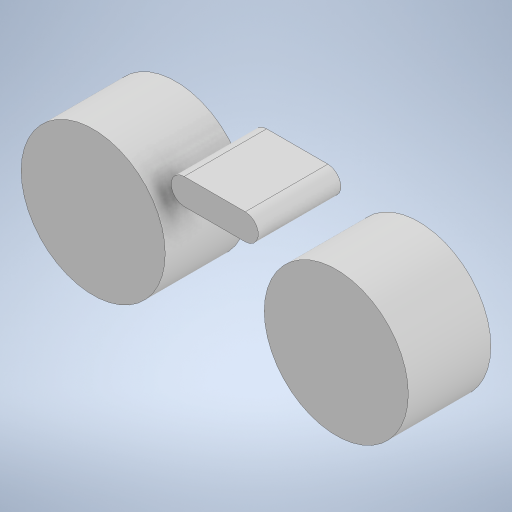
# Autodesk Inventor part: Sonar
Saved by Autodesk Inventor 2024.1 (Build 281209000, 209)
## iProperties
Created: 2024-05-13
Part Number: Sonar
Material: Generic
Document SubType Name: Modeling
Designer: cyan924
Density: 1 g/cm^3
Appearance: Default
Author: cyan924
Autodesk Inventor part; units mm, degrees
(part 1 of 2)
ref_plane "YZ Plane" through (0, 0, 0) normal (1, 0, 0) x (0, 1, 0)
ref_plane "XZ Plane" through (0, 0, 0) normal (0, 1, 0) x (-1, 0, 0)
ref_plane "XY Plane" through (0, 0, 0) normal (0, 0, 1) x (1, 0, 0)
sketch "Sketch1" plane through (0, 0, 0) normal (0, 0, 1) x (1, 0, 0)
  line L0 (-74.4703, -18.8519) -> (-29.4703, -18.8519)
  line L1 (-29.4703, -18.8519) -> (-29.4703, -38.8519)
  line L2 (-29.4703, -38.8519) -> (-74.4703, -38.8519)
  line L3 (-74.4703, -38.8519) -> (-74.4703, -18.8519)
  circle A0 centre (-65.4703, -28.8519) radius 8
  circle A1 centre (-38.4703, -28.8519) radius 8
  arc A2 (-48.5719, -23.254) -> (-48.5719, -20.3658) centre (-48.5719, -21.8099) ccw
  line L4 (-55.3687, -20.3658) -> (-48.5719, -20.3658)
  arc A3 (-55.3687, -20.3658) -> (-55.3687, -23.254) centre (-55.3687, -21.8099) ccw
  line L5 (-48.5719, -23.254) -> (-55.3687, -23.254)
  circle A4 centre (-38.4703, -28.8519) radius 7 construction
  line L6 (-53.2518, -34.5647) -> (-53.3871, -34.5647) construction
  line L7 (-53.3871, -34.5647) -> (-53.3871, -34.4697) construction
  line L8 (-53.3871, -34.4697) -> (-52.7733, -34.4697) construction
  spline S0 degree 3 poles (-52.7733, -34.4697) (-52.7602, -34.4698) (-52.735, -34.47) (-52.6985, -34.4711) (-52.6648, -34.4736) (-52.6337, -34.4764) (-52.6054, -34.4804) (-52.5798, -34.4853) (-52.5569, -34.4908) (-52.5428, -34.4956) (-52.5361, -34.4979) knots 0 0 0 0 0.163445 0.315489 0.456291 0.585864 0.705429 0.813371 0.911718 1 1 1 1 construction
  spline S1 degree 3 poles (-52.5361, -34.4979) (-52.5274, -34.5013) (-52.5103, -34.508) (-52.486, -34.5204) (-52.4632, -34.5344) (-52.4419, -34.5504) (-52.4222, -34.5683) (-52.4038, -34.5876) (-52.3872, -34.609) (-52.3723, -34.6321) (-52.3587, -34.6564) (-52.347, -34.6821) (-52.3373, -34.7092) (-52.3292, -34.7374) (-52.3228, -34.7668) (-52.3185, -34.7974) (-52.3156, -34.8291) (-52.3153, -34.8508) (-52.3152, -34.8617) knots 0 0 0 0 0.061377 0.120918 0.179441 0.23763 0.295967 0.354252 0.413289 0.473845 0.53511 0.596983 0.659861 0.724251 0.789992 0.857734 0.927822 1 1 1 1 construction
  spline S2 degree 3 poles (-52.3152, -34.8617) (-52.3155, -34.8777) (-52.316, -34.9089) (-52.3215, -34.9545) (-52.3302, -34.9977) (-52.3427, -35.0381) (-52.3582, -35.0754) (-52.3759, -35.1093) (-52.3962, -35.1395) (-52.4194, -35.1668) (-52.4469, -35.1914) (-52.4793, -35.2145) (-52.5171, -35.2368) (-52.5449, -35.2498) (-52.5594, -35.2567) knots 0 0 0 0 0.096488 0.188417 0.276865 0.362159 0.443456 0.520182 0.592724 0.662929 0.735428 0.814887 0.903064 1 1 1 1 construction
  line L9 (-52.5594, -35.2567) -> (-52.5594, -35.1617) construction
  spline S3 degree 3 poles (-52.5594, -35.1617) (-52.5473, -35.1541) (-52.5236, -35.1391) (-52.4929, -35.1113) (-52.4668, -35.0805) (-52.4457, -35.0462) (-52.4295, -35.0082) (-52.4182, -34.9661) (-52.4114, -34.9198) (-52.4106, -34.8876) (-52.4101, -34.8708) knots 0 0 0 0 0.124736 0.243843 0.35972 0.474789 0.593462 0.719307 0.853832 1 1 1 1 construction
  spline S4 degree 3 poles (-52.4101, -34.8708) (-52.4106, -34.8543) (-52.4114, -34.8223) (-52.4182, -34.7764) (-52.4295, -34.7345) (-52.4457, -34.6969) (-52.4652, -34.664) (-52.4867, -34.6354) (-52.5113, -34.6124) (-52.5339, -34.5969) (-52.554, -34.5873) (-52.5714, -34.5812) (-52.5909, -34.5762) (-52.6127, -34.572) (-52.6368, -34.5686) (-52.6632, -34.5664) (-52.6917, -34.5648) (-52.7115, -34.5647) (-52.7218, -34.5647) knots 0 0 0 0 0.09818 0.189281 0.274487 0.355219 0.431123 0.501038 0.566565 0.629684 0.662677 0.698735 0.738584 0.782147 0.830394 0.882567 0.939223 1 1 1 1 construction
  line L10 (-52.7218, -34.5647) -> (-52.7619, -34.5647) construction
  spline S5 degree 3 poles (-52.7619, -34.5647) (-52.7504, -34.5743) (-52.7277, -34.5935) (-52.6978, -34.6264) (-52.6724, -34.6626) (-52.6513, -34.7015) (-52.6346, -34.7426) (-52.6224, -34.7852) (-52.6149, -34.8291) (-52.6141, -34.8588) (-52.6137, -34.8738) knots 0 0 0 0 0.126584 0.250941 0.374443 0.499573 0.624733 0.748994 0.873157 1 1 1 1 construction
  spline S6 degree 3 poles (-52.6137, -34.8738) (-52.6139, -34.8826) (-52.6142, -34.9002) (-52.6165, -34.9264) (-52.6209, -34.952) (-52.6265, -34.9773) (-52.634, -35.0021) (-52.6429, -35.0267) (-52.6537, -35.0507) (-52.666, -35.0743) (-52.6797, -35.0968) (-52.6946, -35.1183) (-52.7105, -35.1385) (-52.7276, -35.1574) (-52.746, -35.1748) (-52.7653, -35.191) (-52.7859, -35.2058) (-52.8075, -35.2194) (-52.83, -35.2312) (-52.8531, -35.2416) (-52.8767, -35.2506) (-52.9009, -35.2578) (-52.9256, -35.2633) (-52.9509, -35.2674) (-52.9767, -35.2697) (-52.9941, -35.2701) (-53.0029, -35.2702) knots 0 0 0 0 0.042863 0.085187 0.127219 0.169041 0.210896 0.252856 0.295658 0.338581 0.38149 0.423606 0.465089 0.506333 0.547059 0.587693 0.628691 0.669961 0.711048 0.752006 0.792681 0.833453 0.874196 0.915497 0.95748 1 1 1 1 construction
  spline S7 degree 3 poles (-53.0029, -35.2702) (-53.0117, -35.2701) (-53.0292, -35.2698) (-53.0552, -35.2671) (-53.0808, -35.2632) (-53.1058, -35.2571) (-53.1305, -35.2497) (-53.1546, -35.2406) (-53.1783, -35.2297) (-53.2015, -35.2173) (-53.2239, -35.2033) (-53.2452, -35.1881) (-53.2651, -35.1714) (-53.284, -35.1536) (-53.3017, -35.1345) (-53.318, -35.114) (-53.3333, -35.0924) (-53.3473, -35.0696) (-53.3596, -35.046) (-53.3709, -35.022) (-53.3798, -34.9975) (-53.3877, -34.9729) (-53.3932, -34.9478) (-53.3975, -34.9224) (-53.4001, -34.8967) (-53.4005, -34.8795) (-53.4006, -34.8708) knots 0 0 0 0 0.042034 0.083905 0.125069 0.166158 0.20721 0.248491 0.289878 0.33217 0.374476 0.416225 0.45761 0.499073 0.540553 0.582249 0.62455 0.667433 0.710323 0.752467 0.794065 0.835216 0.876228 0.917446 0.958643 1 1 1 1 construction
  spline S8 degree 3 poles (-53.4006, -34.8708) (-53.4002, -34.8566) (-53.3994, -34.8285) (-53.3931, -34.7872) (-53.3829, -34.7473) (-53.3684, -34.7086) (-53.3486, -34.6708) (-53.3225, -34.6341) (-53.2898, -34.5983) (-53.2648, -34.5762) (-53.2518, -34.5647) knots 0 0 0 0 0.120911 0.238762 0.354755 0.470359 0.589144 0.716329 0.852445 1 1 1 1 construction
  line L11 (-50.2203, -36.6833) -> (-51.2787, -36.6833) construction
  line L12 (-51.2787, -36.6833) -> (-51.2787, -36.0862) construction
  line L13 (-51.2787, -36.0862) -> (-51.1701, -36.0862) construction
  line L14 (-51.1701, -36.0862) -> (-51.1701, -36.5883) construction
  line L15 (-51.1701, -36.5883) -> (-50.8445, -36.5883) construction
  line L16 (-50.8445, -36.5883) -> (-50.8445, -36.0862) construction
  line L17 (-50.8445, -36.0862) -> (-50.7359, -36.0862) construction
  line L18 (-50.7359, -36.0862) -> (-50.7359, -36.5883) construction
  line L19 (-50.7359, -36.5883) -> (-50.3289, -36.5883) construction
  line L20 (-50.3289, -36.5883) -> (-50.3289, -36.0862) construction
  line L21 (-50.3289, -36.0862) -> (-50.2203, -36.0862) construction
  line L22 (-50.2203, -36.0862) -> (-50.2203, -36.6833) construction
  spline S9 degree 3 poles (-51.0073, -35.5176) (-51.007, -35.505) (-51.0065, -35.4797) (-51.0018, -35.4422) (-50.9947, -35.4053) (-50.9843, -35.3696) (-50.9716, -35.3355) (-50.9573, -35.3037) (-50.9411, -35.2746) (-50.923, -35.248) (-50.9024, -35.2238) (-50.8795, -35.2016) (-50.8542, -35.1811) (-50.8355, -35.1695) (-50.826, -35.1636) knots 0 0 0 0 0.091262 0.182067 0.271888 0.362021 0.450031 0.533934 0.613304 0.689893 0.765431 0.841449 0.919739 1 1 1 1 construction
  line L23 (-50.826, -35.1636) -> (-50.7766, -35.2431) construction
  spline S10 degree 3 poles (-50.7766, -35.2431) (-50.7875, -35.2518) (-50.8088, -35.269) (-50.8363, -35.2988) (-50.8599, -35.3305) (-50.8792, -35.3648) (-50.8941, -35.4015) (-50.9046, -35.4405) (-50.9112, -35.4818) (-50.9119, -35.5101) (-50.9123, -35.5246) knots 0 0 0 0 0.128324 0.252584 0.373506 0.493364 0.614609 0.73847 0.865995 1 1 1 1 construction
  spline S11 degree 3 poles (-50.9123, -35.5246) (-50.912, -35.5362) (-50.9114, -35.5591) (-50.9074, -35.5926) (-50.9003, -35.6246) (-50.8909, -35.6551) (-50.8782, -35.6841) (-50.8629, -35.7115) (-50.845, -35.7376) (-50.8243, -35.7617) (-50.8018, -35.7837) (-50.7777, -35.8028) (-50.7527, -35.8194) (-50.7262, -35.8324) (-50.6987, -35.8431) (-50.6698, -35.8501) (-50.6399, -35.8548) (-50.6195, -35.8553) (-50.6091, -35.8556) knots 0 0 0 0 0.069522 0.136921 0.201969 0.265462 0.328248 0.390817 0.45355 0.517542 0.580738 0.641922 0.701597 0.760313 0.818757 0.877718 0.938094 1 1 1 1 construction
  spline S12 degree 3 poles (-50.6091, -35.8556) (-50.5956, -35.855) (-50.5687, -35.854) (-50.5289, -35.8457) (-50.4906, -35.8318) (-50.4538, -35.8131) (-50.4198, -35.7894) (-50.3893, -35.7615) (-50.3628, -35.7295) (-50.3409, -35.6936) (-50.3233, -35.6547) (-50.3108, -35.6131) (-50.3032, -35.5693) (-50.3022, -35.5393) (-50.3017, -35.524) knots 0 0 0 0 0.080524 0.160375 0.240333 0.322539 0.405033 0.486605 0.567872 0.651338 0.736242 0.821532 0.909006 1 1 1 1 construction
  spline S13 degree 3 poles (-50.3017, -35.524) (-50.3021, -35.51) (-50.3029, -35.4824) (-50.3094, -35.4422) (-50.3201, -35.4038) (-50.3349, -35.3674) (-50.3541, -35.333) (-50.3778, -35.3009) (-50.4053, -35.2703) (-50.4266, -35.2523) (-50.4374, -35.2431) knots 0 0 0 0 0.129981 0.255447 0.377298 0.498442 0.619372 0.741857 0.868564 1 1 1 1 construction
  line L24 (-50.4374, -35.2431) -> (-50.3853, -35.1636) construction
  spline S14 degree 3 poles (-50.3853, -35.1636) (-50.3783, -35.1683) (-50.3645, -35.1777) (-50.345, -35.1935) (-50.3268, -35.2104) (-50.3098, -35.2286) (-50.2937, -35.2476) (-50.2793, -35.2683) (-50.2656, -35.2899) (-50.2533, -35.3126) (-50.2423, -35.3363) (-50.2328, -35.3609) (-50.2246, -35.3863) (-50.2182, -35.4125) (-50.213, -35.4396) (-50.2096, -35.4675) (-50.207, -35.4963) (-50.2068, -35.5157) (-50.2068, -35.5255) knots 0 0 0 0 0.059633 0.119069 0.178197 0.236957 0.295932 0.355856 0.416473 0.477742 0.539903 0.602538 0.665422 0.729765 0.794829 0.861827 0.930011 1 1 1 1 construction
  spline S15 degree 3 poles (-50.2068, -35.5255) (-50.207, -35.5405) (-50.2076, -35.5699) (-50.2134, -35.6129) (-50.2221, -35.6541) (-50.2346, -35.6933) (-50.2511, -35.7305) (-50.2708, -35.7659) (-50.2944, -35.7992) (-50.3212, -35.8301) (-50.3503, -35.8583) (-50.3815, -35.8829) (-50.4142, -35.9037) (-50.4485, -35.9209) (-50.4843, -35.9343) (-50.5218, -35.9436) (-50.5607, -35.9495) (-50.5872, -35.9502) (-50.6007, -35.9506) knots 0 0 0 0 0.069569 0.136355 0.201125 0.264488 0.327183 0.389579 0.452173 0.515875 0.579188 0.640132 0.69999 0.75865 0.817794 0.876966 0.937625 1 1 1 1 construction
  spline S16 degree 3 poles (-50.6007, -35.9506) (-50.6098, -35.9504) (-50.6279, -35.9502) (-50.6549, -35.9471) (-50.6815, -35.9432) (-50.7074, -35.9365) (-50.7329, -35.9288) (-50.7579, -35.919) (-50.7824, -35.9075) (-50.8063, -35.8944) (-50.8293, -35.8797) (-50.851, -35.8634) (-50.8717, -35.8462) (-50.8906, -35.8271) (-50.9086, -35.8072) (-50.9252, -35.7857) (-50.9403, -35.7628) (-50.9544, -35.7389) (-50.9669, -35.7139) (-50.9777, -35.688) (-50.9869, -35.6614) (-50.9942, -35.634) (-51.0003, -35.606) (-51.0041, -35.5772) (-51.0068, -35.5477) (-51.0071, -35.5278) (-51.0073, -35.5176) knots 0 0 0 0 0.041291 0.082136 0.122636 0.162831 0.203007 0.243526 0.284173 0.32541 0.366855 0.407551 0.448187 0.488683 0.529015 0.569843 0.61137 0.653238 0.695446 0.737751 0.780043 0.822807 0.865978 0.909595 0.954231 1 1 1 1 construction
  line L25 (-50.2203, -34.9736) -> (-51.3058, -34.9736) construction
  line L26 (-51.3058, -34.9736) -> (-51.3058, -34.8787) construction
  line L27 (-51.3058, -34.8787) -> (-50.8477, -34.8787) construction
  spline S17 degree 3 poles (-50.8477, -34.8787) (-50.8604, -34.8685) (-50.8852, -34.8486) (-50.9176, -34.8152) (-50.9456, -34.7808) (-50.9682, -34.7446) (-50.9859, -34.7067) (-50.9981, -34.6673) (-51.0059, -34.6263) (-51.0068, -34.5985) (-51.0073, -34.5844) knots 0 0 0 0 0.140704 0.273958 0.400629 0.522804 0.641767 0.760002 0.878421 1 1 1 1 construction
  spline S18 degree 3 poles (-51.0073, -34.5844) (-51.0068, -34.5701) (-51.0058, -34.542) (-50.9972, -34.5014) (-50.9837, -34.4631) (-50.9645, -34.4279) (-50.9407, -34.3961) (-50.9131, -34.3683) (-50.8814, -34.3451) (-50.852, -34.3296) (-50.8258, -34.3195) (-50.8034, -34.313) (-50.7784, -34.3076) (-50.7508, -34.3028) (-50.7206, -34.2997) (-50.6878, -34.2971) (-50.6524, -34.2953) (-50.6279, -34.2953) (-50.6153, -34.2952) knots 0 0 0 0 0.077236 0.151245 0.22342 0.29547 0.3669 0.43705 0.506651 0.577825 0.615876 0.658016 0.703748 0.754057 0.808962 0.867901 0.931695 1 1 1 1 construction
  line L28 (-50.6153, -34.2952) -> (-50.2203, -34.2952) construction
  line L29 (-50.2203, -34.2952) -> (-50.2203, -34.3902) construction
  line L30 (-50.2203, -34.3902) -> (-50.5841, -34.3902) construction
  spline S19 degree 3 poles (-50.5841, -34.3902) (-50.5947, -34.3903) (-50.6148, -34.3904) (-50.6436, -34.3907) (-50.6697, -34.3915) (-50.6931, -34.3929) (-50.7138, -34.3942) (-50.7317, -34.3961) (-50.7469, -34.3983) (-50.756, -34.4003) (-50.7601, -34.4012) knots 0 0 0 0 0.178867 0.342142 0.489872 0.622114 0.740055 0.841468 0.928901 1 1 1 1 construction
  spline S20 degree 3 poles (-50.7601, -34.4012) (-50.7721, -34.4047) (-50.7951, -34.4113) (-50.8264, -34.4269) (-50.8532, -34.446) (-50.875, -34.4696) (-50.892, -34.497) (-50.9039, -34.5284) (-50.9112, -34.5635) (-50.9119, -34.5882) (-50.9123, -34.6011) knots 0 0 0 0 0.136267 0.26128 0.379595 0.494345 0.60984 0.729869 0.859203 1 1 1 1 construction
  spline S21 degree 3 poles (-50.9123, -34.6011) (-50.9122, -34.6088) (-50.9119, -34.6239) (-50.909, -34.6463) (-50.9044, -34.6681) (-50.8977, -34.6893) (-50.8895, -34.7098) (-50.8795, -34.7298) (-50.8673, -34.749) (-50.8536, -34.7676) (-50.8385, -34.7849) (-50.8225, -34.801) (-50.8055, -34.8154) (-50.7877, -34.8284) (-50.7689, -34.8397) (-50.7493, -34.8495) (-50.7288, -34.8578) (-50.7146, -34.862) (-50.7075, -34.864) knots 0 0 0 0 0.064023 0.1267 0.189094 0.250549 0.312483 0.374212 0.437823 0.502633 0.567724 0.630558 0.692757 0.754256 0.815111 0.876045 0.937979 1 1 1 1 construction
  spline S22 degree 3 poles (-50.7075, -34.864) (-50.7024, -34.8652) (-50.6912, -34.8678) (-50.6727, -34.8706) (-50.6512, -34.8732) (-50.6267, -34.8753) (-50.5992, -34.8766) (-50.5688, -34.878) (-50.5354, -34.8785) (-50.5121, -34.8786) (-50.5, -34.8787) knots 0 0 0 0 0.075999 0.165611 0.269045 0.387448 0.518827 0.665394 0.825083 1 1 1 1 construction
  line L31 (-50.5, -34.8787) -> (-50.2203, -34.8787) construction
  line L32 (-50.2203, -34.8787) -> (-50.2203, -34.9736) construction
  line L33 (-47.7203, -34.0104) -> (-47.7203, -34.3383) construction
  line L34 (-47.7203, -34.3383) -> (-48.7787, -34.3383) construction
  line L35 (-48.7787, -34.3383) -> (-48.7787, -34.1246) construction
  spline S23 degree 3 poles (-48.7787, -34.1246) (-48.7785, -34.106) (-48.7783, -34.0701) (-48.7766, -34.0182) (-48.7737, -33.9702) (-48.7695, -33.9262) (-48.7643, -33.8862) (-48.7578, -33.8502) (-48.7501, -33.818) (-48.7436, -33.7982) (-48.7405, -33.7888) knots 0 0 0 0 0.164289 0.317406 0.458844 0.589367 0.707831 0.81577 0.91288 1 1 1 1 construction
  spline S24 degree 3 poles (-48.7405, -33.7888) (-48.7358, -33.7766) (-48.7266, -33.7524) (-48.7092, -33.7179) (-48.6895, -33.6853) (-48.6672, -33.655) (-48.6424, -33.6267) (-48.6155, -33.6002) (-48.5857, -33.5761) (-48.5536, -33.554) (-48.5196, -33.5341) (-48.4838, -33.5169) (-48.4464, -33.5025) (-48.4075, -33.4906) (-48.3669, -33.4812) (-48.3246, -33.4748) (-48.2809, -33.4706) (-48.2512, -33.4702) (-48.2361, -33.47) knots 0 0 0 0 0.061546 0.121697 0.181159 0.240077 0.298686 0.357633 0.417592 0.478482 0.540397 0.602336 0.664997 0.728553 0.793646 0.860531 0.929234 1 1 1 1 construction
  spline S25 degree 3 poles (-48.2361, -33.47) (-48.2231, -33.4701) (-48.1973, -33.4705) (-48.1593, -33.4739) (-48.1224, -33.4788) (-48.0869, -33.4863) (-48.0523, -33.4955) (-48.0191, -33.5073) (-47.9869, -33.5208) (-47.9563, -33.5366) (-47.9272, -33.5539) (-47.8998, -33.5723) (-47.8747, -33.5923) (-47.8511, -33.6133) (-47.8298, -33.6358) (-47.8103, -33.6595) (-47.793, -33.6844) (-47.7775, -33.7109) (-47.7637, -33.7391) (-47.7522, -33.7701) (-47.7422, -33.8035) (-47.7343, -33.8398) (-47.7279, -33.8786) (-47.7236, -33.9202) (-47.7207, -33.9644) (-47.7205, -33.9947) (-47.7203, -34.0104) knots 0 0 0 0 0.046084 0.090813 0.134304 0.177036 0.218837 0.260262 0.3011 0.341637 0.381609 0.420148 0.45791 0.494761 0.531219 0.566961 0.602742 0.638232 0.674761 0.713378 0.754425 0.797802 0.843979 0.893064 0.94496 1 1 1 1 construction
  line L36 (-47.7203, -35.3288) -> (-47.7203, -35.4238) construction
  line L37 (-47.7203, -35.4238) -> (-48.7787, -35.4238) construction
  line L38 (-48.7787, -35.4238) -> (-48.7787, -35.4039) construction
  line L39 (-48.7787, -35.4039) -> (-47.9457, -34.7047) construction
  line L40 (-47.9457, -34.7047) -> (-48.7787, -34.7047) construction
  line L41 (-48.7787, -34.7047) -> (-48.7787, -34.6097) construction
  line L42 (-48.7787, -34.6097) -> (-47.7203, -34.6097) construction
  line L43 (-47.7203, -34.6097) -> (-47.7203, -34.6313) construction
  line L44 (-47.7203, -34.6313) -> (-48.5514, -35.3288) construction
  line L45 (-48.5514, -35.3288) -> (-47.7203, -35.3288) construction
  spline S26 degree 3 poles (-48.8058, -36.1843) (-48.8056, -36.1733) (-48.8053, -36.1516) (-48.8029, -36.1192) (-48.799, -36.0874) (-48.7938, -36.056) (-48.7867, -36.0252) (-48.7783, -35.9949) (-48.7684, -35.9649) (-48.7566, -35.9355) (-48.7432, -35.9065) (-48.7281, -35.8776) (-48.7111, -35.8489) (-48.6921, -35.8205) (-48.6715, -35.792) (-48.6486, -35.7641) (-48.6243, -35.736) (-48.6069, -35.7179) (-48.598, -35.7087) knots 0 0 0 0 0.061617 0.122179 0.182216 0.241864 0.30096 0.359969 0.419033 0.478069 0.537993 0.59896 0.661321 0.725248 0.79122 0.858746 0.928318 1 1 1 1 construction
  line L46 (-48.598, -35.7087) -> (-48.5209, -35.7901) construction
  spline S27 degree 3 poles (-48.5209, -35.7901) (-48.5347, -35.8049) (-48.5621, -35.834) (-48.5976, -35.8815) (-48.6283, -35.9309) (-48.6531, -35.9822) (-48.6726, -36.0342) (-48.6867, -36.0858) (-48.6956, -36.1368) (-48.6967, -36.1707) (-48.6972, -36.1874) knots 0 0 0 0 0.136133 0.269021 0.398733 0.527306 0.652311 0.771699 0.887504 1 1 1 1 construction
  spline S28 degree 3 poles (-48.6972, -36.1874) (-48.6971, -36.1977) (-48.6969, -36.2182) (-48.6937, -36.2486) (-48.6891, -36.2787) (-48.6825, -36.3084) (-48.6741, -36.3379) (-48.6635, -36.3669) (-48.6513, -36.3955) (-48.6371, -36.4235) (-48.6215, -36.4506) (-48.6043, -36.4762) (-48.5859, -36.5005) (-48.5659, -36.523) (-48.5446, -36.5438) (-48.5222, -36.5634) (-48.4983, -36.5813) (-48.4731, -36.5973) (-48.4472, -36.6117) (-48.4207, -36.6241) (-48.3938, -36.635) (-48.3665, -36.6432) (-48.339, -36.6502) (-48.311, -36.6551) (-48.2827, -36.6578) (-48.2637, -36.6583) (-48.2542, -36.6585) knots 0 0 0 0 0.04284 0.085568 0.127714 0.170062 0.212779 0.255472 0.298866 0.342848 0.386513 0.429516 0.471868 0.51371 0.555061 0.596513 0.637859 0.67956 0.721068 0.76189 0.801925 0.841812 0.881065 0.920636 0.960103 1 1 1 1 construction
  spline S29 degree 3 poles (-48.2542, -36.6585) (-48.2444, -36.6583) (-48.2249, -36.6578) (-48.1958, -36.6549) (-48.1672, -36.6495) (-48.1389, -36.6423) (-48.111, -36.6331) (-48.0834, -36.6219) (-48.0562, -36.6085) (-48.0297, -36.593) (-48.0038, -36.5759) (-47.9792, -36.5571) (-47.9563, -36.5366) (-47.9345, -36.5147) (-47.9142, -36.4913) (-47.8955, -36.466) (-47.8781, -36.4393) (-47.8623, -36.4112) (-47.8481, -36.382) (-47.8355, -36.3519) (-47.8252, -36.3211) (-47.8167, -36.2896) (-47.8098, -36.2574) (-47.8053, -36.2244) (-47.8021, -36.1909) (-47.8019, -36.1683) (-47.8017, -36.1569) knots 0 0 0 0 0.038996 0.077886 0.116658 0.155425 0.194361 0.234007 0.274295 0.315417 0.356772 0.398061 0.438867 0.479803 0.521246 0.562815 0.605269 0.648388 0.691709 0.735134 0.778356 0.821651 0.865516 0.909726 0.95452 1 1 1 1 construction
  spline S30 degree 3 poles (-47.8017, -36.1569) (-47.802, -36.1432) (-47.8026, -36.1162) (-47.807, -36.0766) (-47.8138, -36.0386) (-47.8239, -36.0022) (-47.8366, -35.9674) (-47.8523, -35.9343) (-47.8709, -35.9028) (-47.8919, -35.873) (-47.9154, -35.8457) (-47.9405, -35.8208) (-47.9675, -35.7992) (-47.9961, -35.7803) (-48.0265, -35.7646) (-48.0586, -35.7518) (-48.0923, -35.742) (-48.1156, -35.7379) (-48.1274, -35.7359) knots 0 0 0 0 0.070637 0.138708 0.204939 0.269469 0.332671 0.395498 0.457967 0.520867 0.583068 0.643278 0.702549 0.760882 0.819471 0.878256 0.938485 1 1 1 1 construction
  line L47 (-48.1274, -35.7359) -> (-48.1274, -36.0886) construction
  line L48 (-48.1274, -36.0886) -> (-48.2359, -36.0886) construction
  line L49 (-48.2359, -36.0886) -> (-48.2359, -35.6409) construction
  spline S31 degree 3 poles (-48.2359, -35.6409) (-48.2157, -35.6414) (-48.1761, -35.6424) (-48.1184, -35.6495) (-48.0638, -35.6609) (-48.0124, -35.6766) (-47.9642, -35.6968) (-47.9192, -35.7214) (-47.8777, -35.7508) (-47.8393, -35.7839) (-47.805, -35.821) (-47.7749, -35.8613) (-47.7495, -35.9046) (-47.7289, -35.951) (-47.7128, -36.0003) (-47.7014, -36.0526) (-47.6945, -36.1079) (-47.6936, -36.1458) (-47.6932, -36.1652) knots 0 0 0 0 0.071272 0.139493 0.204635 0.267406 0.328446 0.388397 0.447734 0.507392 0.566768 0.625478 0.684067 0.743248 0.804033 0.866499 0.931723 1 1 1 1 construction
  spline S32 degree 3 poles (-47.6932, -36.1652) (-47.6934, -36.1771) (-47.6937, -36.2007) (-47.6961, -36.2355) (-47.6998, -36.2693) (-47.7054, -36.3022) (-47.7123, -36.3342) (-47.7211, -36.3653) (-47.7313, -36.3954) (-47.7429, -36.4247) (-47.7563, -36.4529) (-47.7712, -36.4802) (-47.7875, -36.5065) (-47.8055, -36.5319) (-47.8251, -36.5564) (-47.8463, -36.5799) (-47.869, -36.6025) (-47.8852, -36.6166) (-47.8933, -36.6238) knots 0 0 0 0 0.069237 0.136557 0.202094 0.266464 0.329769 0.391879 0.453271 0.514115 0.57439 0.634142 0.693923 0.754152 0.81447 0.875661 0.937348 1 1 1 1 construction
  spline S33 degree 3 poles (-47.8933, -36.6238) (-47.9062, -36.6341) (-47.9318, -36.6546) (-47.9728, -36.681) (-48.0153, -36.7035) (-48.0593, -36.7217) (-48.1049, -36.736) (-48.1519, -36.7462) (-48.2004, -36.7522) (-48.2333, -36.7531) (-48.2499, -36.7535) knots 0 0 0 0 0.127896 0.253668 0.376738 0.499344 0.621999 0.745699 0.871345 1 1 1 1 construction
  spline S34 degree 3 poles (-48.2499, -36.7535) (-48.2624, -36.7533) (-48.2871, -36.753) (-48.3238, -36.7491) (-48.3599, -36.7436) (-48.3953, -36.7354) (-48.43, -36.7251) (-48.4641, -36.7122) (-48.4976, -36.6972) (-48.5302, -36.6798) (-48.5616, -36.6605) (-48.5915, -36.6394) (-48.6194, -36.6165) (-48.6456, -36.5917) (-48.6703, -36.5655) (-48.6929, -36.5374) (-48.714, -36.5077) (-48.733, -36.4763) (-48.7502, -36.4436) (-48.7651, -36.4097) (-48.7775, -36.3746) (-48.7881, -36.3387) (-48.7958, -36.3015) (-48.8015, -36.2634) (-48.8053, -36.2242) (-48.8056, -36.1977) (-48.8058, -36.1843) knots 0 0 0 0 0.04204 0.083545 0.124644 0.165305 0.206173 0.246974 0.288333 0.32999 0.371802 0.412742 0.453464 0.493833 0.534375 0.574947 0.615887 0.657246 0.699003 0.740483 0.782323 0.824565 0.86704 0.910499 0.954619 1 1 1 1 construction
  spline S35 degree 3 poles (-50.8792, -33.9993) (-50.8895, -33.9894) (-50.9097, -33.9702) (-50.9356, -33.9377) (-50.9579, -33.9037) (-50.9759, -33.8675) (-50.9901, -33.8295) (-50.9999, -33.7895) (-51.0064, -33.7477) (-51.007, -33.7191) (-51.0073, -33.7046) knots 0 0 0 0 0.128498 0.252713 0.374819 0.496436 0.617911 0.741288 0.8687 1 1 1 1 construction
  spline S36 degree 3 poles (-51.0073, -33.7046) (-51.007, -33.6901) (-51.0064, -33.6616) (-50.9999, -33.6199) (-50.99, -33.5802) (-50.9763, -33.5421) (-50.958, -33.5063) (-50.9361, -33.4722) (-50.9101, -33.4399) (-50.8901, -33.4206) (-50.8799, -33.4107) knots 0 0 0 0 0.131751 0.258332 0.382134 0.503804 0.624693 0.746871 0.871514 1 1 1 1 construction
  spline S37 degree 3 poles (-50.8799, -33.4107) (-50.8701, -33.4023) (-50.8508, -33.3855) (-50.8196, -33.364) (-50.7872, -33.3455) (-50.7532, -33.3307) (-50.718, -33.319) (-50.6815, -33.3107) (-50.6436, -33.3057) (-50.6179, -33.3051) (-50.6049, -33.3047) knots 0 0 0 0 0.128157 0.253834 0.376506 0.498534 0.621368 0.744565 0.870634 1 1 1 1 construction
  spline S38 degree 3 poles (-50.6049, -33.3047) (-50.5918, -33.305) (-50.5659, -33.3056) (-50.5278, -33.3112) (-50.4909, -33.3198) (-50.4552, -33.3321) (-50.4208, -33.348) (-50.3877, -33.3673) (-50.3559, -33.3902) (-50.3257, -33.4162) (-50.2978, -33.445) (-50.2735, -33.4762) (-50.2527, -33.5092) (-50.236, -33.5444) (-50.2227, -33.5816) (-50.2135, -33.6209) (-50.2078, -33.6621) (-50.2071, -33.6902) (-50.2068, -33.7046) knots 0 0 0 0 0.062416 0.123337 0.183265 0.243172 0.302898 0.363774 0.425605 0.489659 0.553785 0.616222 0.677854 0.739517 0.802097 0.865866 0.931508 1 1 1 1 construction
  spline S39 degree 3 poles (-50.2068, -33.7046) (-50.2071, -33.719) (-50.2079, -33.7473) (-50.2134, -33.7886) (-50.2227, -33.8279) (-50.236, -33.8652) (-50.2527, -33.9006) (-50.2735, -33.9338) (-50.2978, -33.965) (-50.3257, -33.9938) (-50.3559, -34.0198) (-50.3877, -34.0427) (-50.4208, -34.062) (-50.4552, -34.0779) (-50.4909, -34.0902) (-50.5278, -34.0988) (-50.5659, -34.1044) (-50.5918, -34.105) (-50.6049, -34.1053) knots 0 0 0 0 0.068742 0.134635 0.198324 0.260825 0.322714 0.384555 0.446913 0.510958 0.574931 0.636685 0.697483 0.757134 0.816966 0.876818 0.937663 1 1 1 1 construction
  spline S40 degree 3 poles (-50.6049, -34.1053) (-50.6179, -34.1049) (-50.6435, -34.1043) (-50.6813, -34.0993) (-50.7177, -34.0911) (-50.7527, -34.0792) (-50.7866, -34.0644) (-50.8191, -34.0461) (-50.8502, -34.0244) (-50.8695, -34.0077) (-50.8792, -33.9993) knots 0 0 0 0 0.128922 0.255244 0.378688 0.500432 0.622705 0.746235 0.871586 1 1 1 1 construction
  line L50 (-52.6137, -35.5552) -> (-53.3871, -35.5552) construction
  line L51 (-53.3871, -35.5552) -> (-53.3871, -35.4602) construction
  line L52 (-53.3871, -35.4602) -> (-52.6137, -35.4602) construction
  line L53 (-52.6137, -35.4602) -> (-52.6137, -35.5552) construction
  spline S41 degree 3 poles (-53.6309, -35.5959) (-53.6364, -35.5956) (-53.6471, -35.5949) (-53.6626, -35.5897) (-53.6768, -35.5816) (-53.6892, -35.5703) (-53.6995, -35.5568) (-53.7072, -35.5417) (-53.7119, -35.5253) (-53.7124, -35.5139) (-53.7127, -35.5081) knots 0 0 0 0 0.12329 0.242149 0.363437 0.489745 0.618115 0.744894 0.868932 1 1 1 1 construction
  spline S42 degree 3 poles (-53.7127, -35.5081) (-53.7124, -35.5022) (-53.7119, -35.4907) (-53.7073, -35.474) (-53.6995, -35.4588) (-53.6891, -35.4453) (-53.6769, -35.4338) (-53.6626, -35.4257) (-53.6471, -35.4204) (-53.6364, -35.4198) (-53.6309, -35.4195) knots 0 0 0 0 0.131899 0.258284 0.384341 0.51198 0.638632 0.75923 0.877412 1 1 1 1 construction
  spline S43 degree 3 poles (-53.6309, -35.4195) (-53.6255, -35.4198) (-53.615, -35.4205) (-53.5998, -35.4256) (-53.5857, -35.4338) (-53.5735, -35.4453) (-53.5631, -35.4588) (-53.5553, -35.474) (-53.5507, -35.4907) (-53.5502, -35.5022) (-53.5499, -35.5081) knots 0 0 0 0 0.120162 0.237546 0.357497 0.484917 0.613329 0.74015 0.867301 1 1 1 1 construction
  spline S44 degree 3 poles (-53.5499, -35.5081) (-53.5502, -35.5139) (-53.5507, -35.5253) (-53.5554, -35.5417) (-53.5631, -35.5568) (-53.5734, -35.5703) (-53.5858, -35.5816) (-53.5998, -35.5897) (-53.615, -35.5949) (-53.6255, -35.5956) (-53.6309, -35.5959) knots 0 0 0 0 0.131867 0.256661 0.384213 0.513365 0.640443 0.761085 0.879146 1 1 1 1 construction
  line L54 (-52.6137, -36.0165) -> (-53.3871, -36.0165) construction
  line L55 (-53.3871, -36.0165) -> (-53.3871, -35.9215) construction
  line L56 (-53.3871, -35.9215) -> (-53.2732, -35.9215) construction
  spline S45 degree 3 poles (-53.2732, -35.9215) (-53.2838, -35.9145) (-53.3041, -35.9011) (-53.3309, -35.8787) (-53.3533, -35.8561) (-53.371, -35.8325) (-53.3843, -35.8083) (-53.3937, -35.7836) (-53.3995, -35.7583) (-53.4003, -35.7414) (-53.4006, -35.7328) knots 0 0 0 0 0.160011 0.306021 0.438854 0.560992 0.675734 0.786178 0.892874 1 1 1 1 construction
  spline S46 degree 3 poles (-53.4006, -35.7328) (-53.4003, -35.7262) (-53.3995, -35.7127) (-53.3943, -35.6921) (-53.386, -35.6709) (-53.3782, -35.6573) (-53.3741, -35.6502) knots 0 0 0 0 0.225278 0.463523 0.720324 1 1 1 1 construction
  line L57 (-53.3741, -35.6502) -> (-53.2919, -35.7023) construction
  spline S47 degree 3 poles (-53.2919, -35.7023) (-53.2939, -35.7069) (-53.2978, -35.7156) (-53.3024, -35.7282) (-53.3051, -35.7399) (-53.3055, -35.7474) (-53.3057, -35.7509) knots 0 0 0 0 0.295139 0.56023 0.794983 1 1 1 1 construction
  spline S48 degree 3 poles (-53.3057, -35.7509) (-53.3052, -35.7585) (-53.3041, -35.774) (-53.2959, -35.7968) (-53.2831, -35.8191) (-53.2684, -35.8366) (-53.2543, -35.8502) (-53.242, -35.86) (-53.2281, -35.8688) (-53.2131, -35.8773) (-53.1966, -35.8852) (-53.1786, -35.8923) (-53.1593, -35.8989) (-53.1459, -35.9027) (-53.139, -35.9046) knots 0 0 0 0 0.093777 0.191278 0.294662 0.409747 0.471345 0.53582 0.603222 0.674199 0.748603 0.828338 0.912068 1 1 1 1 construction
  spline S49 degree 3 poles (-53.139, -35.9046) (-53.1329, -35.906) (-53.1192, -35.9092) (-53.0965, -35.9122) (-53.0695, -35.9153) (-53.0385, -35.9174) (-53.0031, -35.9194) (-52.9637, -35.9205) (-52.92, -35.9215) (-52.8896, -35.9215) (-52.8736, -35.9215) knots 0 0 0 0 0.070855 0.157726 0.258598 0.375889 0.508164 0.657032 0.820176 1 1 1 1 construction
  line L58 (-52.8736, -35.9215) -> (-52.6137, -35.9215) construction
  line L59 (-52.6137, -35.9215) -> (-52.6137, -36.0165) construction
  line L60 (-53.5635, -36.4778) -> (-53.5635, -36.7085) construction
  line L61 (-53.5635, -36.7085) -> (-53.672, -36.7085) construction
  line L62 (-53.672, -36.7085) -> (-53.672, -36.1522) construction
  line L63 (-53.672, -36.1522) -> (-53.5635, -36.1522) construction
  line L64 (-53.5635, -36.1522) -> (-53.5635, -36.3829) construction
  line L65 (-53.5635, -36.3829) -> (-52.6137, -36.3829) construction
  line L66 (-52.6137, -36.3829) -> (-52.6137, -36.4778) construction
  line L67 (-52.6137, -36.4778) -> (-53.5635, -36.4778) construction
  line L68 (-55.1196, -36.5888) -> (-56.1779, -36.9009) construction
  line L69 (-56.1779, -36.9009) -> (-56.1779, -36.8269) construction
  line L70 (-56.1779, -36.8269) -> (-55.3475, -36.582) construction
  line L71 (-55.3475, -36.582) -> (-56.1779, -36.3371) construction
  line L72 (-56.1779, -36.3371) -> (-56.1779, -36.2632) construction
  line L73 (-56.1779, -36.2632) -> (-55.1196, -36.5752) construction
  line L74 (-55.1196, -36.5752) -> (-55.1196, -36.5888) construction
  spline S50 degree 3 poles (-56.2051, -35.5953) (-56.2049, -35.587) (-56.2046, -35.5705) (-56.2018, -35.5461) (-56.1971, -35.5224) (-56.1907, -35.4992) (-56.1827, -35.4767) (-56.1726, -35.4547) (-56.1608, -35.4334) (-56.1471, -35.4127) (-56.1318, -35.3928) (-56.1151, -35.3737) (-56.0968, -35.3557) (-56.077, -35.3385) (-56.0558, -35.3222) (-56.0332, -35.3068) (-56.0091, -35.2924) (-55.9922, -35.2838) (-55.9837, -35.2794) knots 0 0 0 0 0.061412 0.121093 0.180462 0.239266 0.297837 0.356726 0.416795 0.477241 0.538829 0.601118 0.664013 0.728161 0.793808 0.86046 0.929504 1 1 1 1 construction
  line L75 (-55.9837, -35.2794) -> (-55.9201, -35.3363) construction
  spline S51 degree 3 poles (-55.9201, -35.3363) (-55.9339, -35.3443) (-55.9606, -35.3599) (-55.9964, -35.3877) (-56.027, -35.4177) (-56.0523, -35.4501) (-56.072, -35.4846) (-56.0862, -35.5209) (-56.095, -35.5589) (-56.096, -35.585) (-56.0965, -35.5981) knots 0 0 0 0 0.143848 0.279439 0.407624 0.53045 0.649366 0.765173 0.881623 1 1 1 1 construction
  spline S52 degree 3 poles (-56.0965, -35.5981) (-56.0964, -35.6053) (-56.0961, -35.6197) (-56.0929, -35.6411) (-56.0883, -35.6621) (-56.0817, -35.6827) (-56.0731, -35.7028) (-56.063, -35.7227) (-56.0506, -35.7419) (-56.0366, -35.7608) (-56.0211, -35.7789) (-56.0039, -35.7959) (-55.9858, -35.8121) (-55.9661, -35.8269) (-55.9453, -35.841) (-55.9232, -35.8539) (-55.8999, -35.8658) (-55.8669, -35.8803) (-55.8228, -35.8951) (-55.7673, -35.908) (-55.7085, -35.9158) (-55.6683, -35.9167) (-55.6477, -35.9172) knots 0 0 0 0 0.035491 0.070944 0.105865 0.141271 0.17711 0.213498 0.251017 0.289542 0.328988 0.368325 0.408228 0.448422 0.489502 0.531423 0.574339 0.618397 0.708777 0.802307 0.898737 1 1 1 1 construction
  spline S53 degree 3 poles (-55.6477, -35.9172) (-55.6321, -35.9169) (-55.6015, -35.9163) (-55.5565, -35.912) (-55.5136, -35.9048) (-55.4726, -35.8949) (-55.4336, -35.882) (-55.3966, -35.866) (-55.3615, -35.8473) (-55.3288, -35.8261) (-55.299, -35.8025) (-55.2727, -35.7773) (-55.2507, -35.7503) (-55.2325, -35.722) (-55.2183, -35.6921) (-55.2084, -35.6606) (-55.2019, -35.6276) (-55.2013, -35.605) (-55.201, -35.5936) knots 0 0 0 0 0.076489 0.149807 0.220668 0.289383 0.356113 0.421658 0.486347 0.550345 0.612636 0.67184 0.728137 0.782739 0.836281 0.889669 0.944218 1 1 1 1 construction
  spline S54 degree 3 poles (-55.201, -35.5936) (-55.2015, -35.581) (-55.2025, -35.556) (-55.2112, -35.5195) (-55.2251, -35.4846) (-55.2446, -35.4512) (-55.2698, -35.4196) (-55.3005, -35.3899) (-55.3365, -35.3615) (-55.3634, -35.3449) (-55.3774, -35.3363) knots 0 0 0 0 0.115519 0.228411 0.341993 0.458888 0.581001 0.710531 0.849729 1 1 1 1 construction
  line L76 (-55.3774, -35.3363) -> (-55.3144, -35.2794) construction
  spline S55 degree 3 poles (-55.3144, -35.2794) (-55.3058, -35.2841) (-55.2889, -35.2931) (-55.2644, -35.3076) (-55.2418, -35.3235) (-55.2204, -35.3397) (-55.2008, -35.3572) (-55.1824, -35.3752) (-55.1657, -35.3943) (-55.1504, -35.414) (-55.1367, -35.4344) (-55.1249, -35.4555) (-55.1149, -35.4773) (-55.1064, -35.4994) (-55.1005, -35.5225) (-55.0957, -35.5459) (-55.0929, -35.57) (-55.0926, -35.5863) (-55.0924, -35.5945) knots 0 0 0 0 0.071835 0.141733 0.209538 0.275317 0.339938 0.402959 0.465373 0.526672 0.586806 0.646541 0.705074 0.762964 0.821246 0.880223 0.939506 1 1 1 1 construction
  spline S56 degree 3 poles (-55.0924, -35.5945) (-55.0925, -35.6023) (-55.0927, -35.6177) (-55.0953, -35.6404) (-55.0987, -35.6626) (-55.1039, -35.6841) (-55.1102, -35.7051) (-55.1183, -35.7253) (-55.1277, -35.745) (-55.1384, -35.7641) (-55.1509, -35.7824) (-55.1646, -35.8002) (-55.1799, -35.8173) (-55.1966, -35.8337) (-55.2146, -35.8497) (-55.2342, -35.8649) (-55.2551, -35.8796) (-55.27, -35.8886) (-55.2775, -35.8932) knots 0 0 0 0 0.063148 0.124874 0.185914 0.245488 0.304302 0.363551 0.422073 0.481436 0.540963 0.601914 0.664105 0.727002 0.792053 0.859094 0.928344 1 1 1 1 construction
  spline S57 degree 3 poles (-55.2775, -35.8932) (-55.2908, -35.9006) (-55.3175, -35.9154) (-55.3598, -35.9338) (-55.404, -35.9498) (-55.4503, -35.9628) (-55.4986, -35.9726) (-55.5489, -35.9799) (-55.6013, -35.9841) (-55.6368, -35.9847) (-55.6549, -35.985) knots 0 0 0 0 0.115614 0.233006 0.352296 0.473908 0.599503 0.728676 0.861834 1 1 1 1 construction
  spline S58 degree 3 poles (-55.6549, -35.985) (-55.6739, -35.9847) (-55.7113, -35.9841) (-55.7661, -35.9787) (-55.8186, -35.97) (-55.8688, -35.958) (-55.9167, -35.9422) (-55.9623, -35.9232) (-56.0057, -35.9006) (-56.0462, -35.8747) (-56.0834, -35.8465) (-56.1158, -35.8159) (-56.1434, -35.7836) (-56.1659, -35.7494) (-56.1837, -35.7134) (-56.1959, -35.6755) (-56.2036, -35.636) (-56.2046, -35.609) (-56.2051, -35.5953) knots 0 0 0 0 0.076323 0.149835 0.220843 0.289698 0.356871 0.422972 0.48792 0.552826 0.615732 0.675113 0.731253 0.78592 0.838938 0.891762 0.945159 1 1 1 1 construction
  spline S59 degree 3 poles (-56.2051, -34.5981) (-56.2049, -34.5897) (-56.2046, -34.5733) (-56.2018, -34.5489) (-56.1971, -34.5251) (-56.1907, -34.502) (-56.1827, -34.4794) (-56.1726, -34.4574) (-56.1608, -34.4361) (-56.1471, -34.4154) (-56.1318, -34.3956) (-56.1151, -34.3764) (-56.0968, -34.3584) (-56.077, -34.3412) (-56.0558, -34.3249) (-56.0332, -34.3096) (-56.0091, -34.2952) (-55.9922, -34.2865) (-55.9837, -34.2822) knots 0 0 0 0 0.061412 0.121093 0.180462 0.239266 0.297837 0.356726 0.416795 0.477241 0.538829 0.601118 0.664013 0.728161 0.793808 0.86046 0.929504 1 1 1 1 construction
  line L77 (-55.9837, -34.2822) -> (-55.9201, -34.339) construction
  spline S60 degree 3 poles (-55.9201, -34.339) (-55.9339, -34.347) (-55.9606, -34.3626) (-55.9964, -34.3904) (-56.027, -34.4204) (-56.0523, -34.4528) (-56.072, -34.4873) (-56.0862, -34.5236) (-56.095, -34.5617) (-56.096, -34.5877) (-56.0965, -34.6008) knots 0 0 0 0 0.143848 0.279439 0.407624 0.53045 0.649366 0.765173 0.881623 1 1 1 1 construction
  spline S61 degree 3 poles (-56.0965, -34.6008) (-56.0964, -34.608) (-56.0961, -34.6225) (-56.0929, -34.6438) (-56.0883, -34.6648) (-56.0817, -34.6854) (-56.0731, -34.7055) (-56.063, -34.7254) (-56.0506, -34.7447) (-56.0366, -34.7635) (-56.0211, -34.7817) (-56.0039, -34.7986) (-55.9858, -34.8148) (-55.9661, -34.8296) (-55.9453, -34.8437) (-55.9232, -34.8566) (-55.8999, -34.8685) (-55.8669, -34.883) (-55.8228, -34.8978) (-55.7673, -34.9107) (-55.7085, -34.9185) (-55.6683, -34.9194) (-55.6477, -34.9199) knots 0 0 0 0 0.035491 0.070944 0.105865 0.141271 0.17711 0.213498 0.251017 0.289542 0.328988 0.368325 0.408228 0.448422 0.489502 0.531423 0.574339 0.618397 0.708777 0.802307 0.898737 1 1 1 1 construction
  spline S62 degree 3 poles (-55.6477, -34.9199) (-55.6321, -34.9196) (-55.6015, -34.919) (-55.5565, -34.9148) (-55.5136, -34.9075) (-55.4726, -34.8977) (-55.4336, -34.8847) (-55.3966, -34.8687) (-55.3615, -34.8501) (-55.3288, -34.8288) (-55.299, -34.8052) (-55.2727, -34.7801) (-55.2507, -34.7531) (-55.2325, -34.7248) (-55.2183, -34.6948) (-55.2084, -34.6633) (-55.2019, -34.6303) (-55.2013, -34.6078) (-55.201, -34.5964) knots 0 0 0 0 0.076489 0.149807 0.220668 0.289383 0.356113 0.421658 0.486347 0.550345 0.612636 0.67184 0.728137 0.782739 0.836281 0.889669 0.944218 1 1 1 1 construction
  spline S63 degree 3 poles (-55.201, -34.5964) (-55.2015, -34.5837) (-55.2025, -34.5588) (-55.2112, -34.5222) (-55.2251, -34.4873) (-55.2446, -34.454) (-55.2698, -34.4224) (-55.3005, -34.3926) (-55.3365, -34.3643) (-55.3634, -34.3476) (-55.3774, -34.339) knots 0 0 0 0 0.115519 0.228411 0.341993 0.458888 0.581001 0.710531 0.849729 1 1 1 1 construction
  line L78 (-55.3774, -34.339) -> (-55.3144, -34.2822) construction
  spline S64 degree 3 poles (-55.3144, -34.2822) (-55.3058, -34.2868) (-55.2889, -34.2959) (-55.2644, -34.3103) (-55.2418, -34.3262) (-55.2204, -34.3424) (-55.2008, -34.3599) (-55.1824, -34.3779) (-55.1657, -34.397) (-55.1504, -34.4167) (-55.1367, -34.4372) (-55.1249, -34.4583) (-55.1149, -34.48) (-55.1064, -34.5021) (-55.1005, -34.5252) (-55.0957, -34.5486) (-55.0929, -34.5728) (-55.0926, -34.589) (-55.0924, -34.5972) knots 0 0 0 0 0.071835 0.141733 0.209538 0.275317 0.339938 0.402959 0.465373 0.526672 0.586806 0.646541 0.705074 0.762964 0.821246 0.880223 0.939506 1 1 1 1 construction
  spline S65 degree 3 poles (-55.0924, -34.5972) (-55.0925, -34.605) (-55.0927, -34.6204) (-55.0953, -34.6432) (-55.0987, -34.6654) (-55.1039, -34.6869) (-55.1102, -34.7078) (-55.1183, -34.728) (-55.1277, -34.7477) (-55.1384, -34.7668) (-55.1509, -34.7851) (-55.1646, -34.8029) (-55.1799, -34.8201) (-55.1966, -34.8365) (-55.2146, -34.8524) (-55.2342, -34.8676) (-55.2551, -34.8823) (-55.27, -34.8913) (-55.2775, -34.8959) knots 0 0 0 0 0.063148 0.124874 0.185914 0.245488 0.304302 0.363551 0.422073 0.481436 0.540963 0.601914 0.664105 0.727002 0.792053 0.859094 0.928344 1 1 1 1 construction
  spline S66 degree 3 poles (-55.2775, -34.8959) (-55.2908, -34.9033) (-55.3175, -34.9181) (-55.3598, -34.9365) (-55.404, -34.9525) (-55.4503, -34.9655) (-55.4986, -34.9753) (-55.5489, -34.9826) (-55.6013, -34.9869) (-55.6368, -34.9874) (-55.6549, -34.9877) knots 0 0 0 0 0.115614 0.233006 0.352296 0.473908 0.599503 0.728676 0.861834 1 1 1 1 construction
  spline S67 degree 3 poles (-55.6549, -34.9877) (-55.6739, -34.9874) (-55.7113, -34.9869) (-55.7661, -34.9814) (-55.8186, -34.9728) (-55.8688, -34.9608) (-55.9167, -34.9449) (-55.9623, -34.926) (-56.0057, -34.9033) (-56.0462, -34.8775) (-56.0834, -34.8492) (-56.1158, -34.8186) (-56.1434, -34.7863) (-56.1659, -34.7521) (-56.1837, -34.7161) (-56.1959, -34.6783) (-56.2036, -34.6387) (-56.2046, -34.6117) (-56.2051, -34.5981) knots 0 0 0 0 0.076323 0.149835 0.220843 0.289698 0.356871 0.422972 0.48792 0.552826 0.615732 0.675113 0.731253 0.78592 0.838938 0.891762 0.945159 1 1 1 1 construction
  circle A5 centre (-72.9703, -37.3519) radius 1.25 construction
  circle A6 centre (-30.9703, -37.3519) radius 1.25 construction
  circle A7 centre (-30.9703, -20.3519) radius 1.25 construction
  circle A8 centre (-72.9703, -20.3519) radius 1.25 construction
  line L79 (-29.4703, -38.8519) -> (-29.4703, -18.8519) construction
  line L80 (-29.4703, -18.8519) -> (-74.4703, -18.8519) construction
  line L81 (-74.4703, -18.8519) -> (-74.4703, -38.8519) construction
  line L82 (-74.4703, -38.8519) -> (-29.4703, -38.8519) construction
  line L83 (-47.688, -25.8917) -> (-47.0717, -23.9989) construction
  line L84 (-47.0717, -23.9989) -> (-47.0469, -23.9989) construction
  line L85 (-47.0469, -23.9989) -> (-47.0469, -25.6475) construction
  line L86 (-47.0469, -25.6475) -> (-46.8942, -25.6475) construction
  line L87 (-46.8942, -25.6475) -> (-46.8942, -25.8917) construction
  line L88 (-46.8942, -25.8917) -> (-47.0469, -25.8917) construction
  line L89 (-47.0469, -25.8917) -> (-47.0469, -26.4412) construction
  line L90 (-47.0469, -26.4412) -> (-47.169, -26.4412) construction
  line L91 (-47.169, -26.4412) -> (-47.169, -25.8917) construction
  line L92 (-47.169, -25.8917) -> (-47.688, -25.8917) construction
  line L93 (-50.6981, -26.4412) -> (-50.6981, -24.06) construction
  line L94 (-50.6981, -24.06) -> (-50.4549, -24.06) construction
  spline S68 degree 3 poles (-50.4549, -24.06) (-50.4386, -24.0601) (-50.4075, -24.0603) (-50.3628, -24.0614) (-50.3222, -24.0646) (-50.2857, -24.0675) (-50.2535, -24.0725) (-50.225, -24.0774) (-50.2007, -24.0839) (-50.1863, -24.0897) (-50.1796, -24.0924) knots 0 0 0 0 0.174617 0.335612 0.481481 0.612132 0.729789 0.832528 0.923062 1 1 1 1 construction
  spline S69 degree 3 poles (-50.1796, -24.0924) (-50.1706, -24.0968) (-50.1523, -24.1056) (-50.127, -24.1237) (-50.1031, -24.1449) (-50.0799, -24.1691) (-50.0593, -24.1979) (-50.0385, -24.229) (-50.02, -24.2644) (-49.9962, -24.3165) (-49.9706, -24.3886) (-49.9503, -24.4834) (-49.9371, -24.587) (-49.9357, -24.6592) (-49.9349, -24.6968) knots 0 0 0 0 0.044006 0.089111 0.135588 0.184459 0.235818 0.290786 0.34854 0.410681 0.542441 0.683297 0.835197 1 1 1 1 construction
  spline S70 degree 3 poles (-49.9349, -24.6968) (-49.9354, -24.7284) (-49.9363, -24.7898) (-49.9457, -24.8789) (-49.9601, -24.9623) (-49.9809, -25.0393) (-50.0068, -25.1089) (-50.0376, -25.1704) (-50.0746, -25.2224) (-50.1166, -25.2662) (-50.1661, -25.3008) (-50.2243, -25.3243) (-50.2903, -25.3394) (-50.3373, -25.3412) (-50.3618, -25.3422) knots 0 0 0 0 0.108599 0.210585 0.306992 0.39856 0.483663 0.561484 0.633835 0.701724 0.768755 0.839164 0.915783 1 1 1 1 construction
  line L95 (-50.3618, -25.3422) -> (-49.9349, -26.4412) construction
  line L96 (-49.9349, -26.4412) -> (-50.0895, -26.4412) construction
  line L97 (-50.0895, -26.4412) -> (-50.5164, -25.3422) construction
  line L98 (-50.5164, -25.3422) -> (-50.576, -25.3422) construction
  line L99 (-50.576, -25.3422) -> (-50.576, -26.4412) construction
  line L100 (-50.576, -26.4412) -> (-50.6981, -26.4412) construction
  line L101 (-53.403, -25.6475) -> (-53.403, -25.4032) construction
  line L102 (-53.403, -25.4032) -> (-52.9451, -25.4032) construction
  line L103 (-52.9451, -25.4032) -> (-52.9451, -25.6475) construction
  line L104 (-52.9451, -25.6475) -> (-53.403, -25.6475) construction
  line L105 (-56.9321, -26.4412) -> (-56.9321, -24.06) construction
  line L106 (-56.9321, -24.06) -> (-56.81, -24.06) construction
  line L107 (-56.81, -24.06) -> (-56.81, -25.0369) construction
  line L108 (-56.81, -25.0369) -> (-56.23, -25.0369) construction
  line L109 (-56.23, -25.0369) -> (-56.23, -24.06) construction
  line L110 (-56.23, -24.06) -> (-56.1079, -24.06) construction
  line L111 (-56.1079, -24.06) -> (-56.1079, -26.4412) construction
  line L112 (-56.1079, -26.4412) -> (-56.23, -26.4412) construction
  line L113 (-56.23, -26.4412) -> (-56.23, -25.2811) construction
  line L114 (-56.23, -25.2811) -> (-56.81, -25.2811) construction
  line L115 (-56.81, -25.2811) -> (-56.81, -26.4412) construction
  line L116 (-56.81, -26.4412) -> (-56.9321, -26.4412) construction
  arc A9 (-48.5719, -22.254) -> (-48.5719, -21.3658) centre (-48.5719, -21.8099) ccw construction
  line L117 (-48.5719, -22.254) -> (-55.3687, -22.254) construction
  arc A10 (-55.3687, -21.3658) -> (-55.3687, -22.254) centre (-55.3687, -21.8099) ccw construction
  line L118 (-55.3687, -21.3658) -> (-48.5719, -21.3658) construction
  spline S71 degree 3 poles (-54.6185, -23.9989) (-54.6048, -23.9992) (-54.5776, -23.9999) (-54.5373, -24.0063) (-54.4981, -24.0168) (-54.4601, -24.0315) (-54.4226, -24.0493) (-54.3869, -24.0728) (-54.3515, -24.0993) (-54.3177, -24.1302) (-54.2848, -24.1643) (-54.2537, -24.2022) (-54.2245, -24.2435) (-54.1952, -24.2871) (-54.1696, -24.3353) (-54.144, -24.3859) (-54.1202, -24.44) (-54.1062, -24.4777) (-54.0991, -24.4969) knots 0 0 0 0 0.053533 0.106387 0.159178 0.211724 0.265674 0.321043 0.378748 0.438185 0.500194 0.563807 0.629731 0.698028 0.768993 0.842684 0.920089 1 1 1 1 construction
  line L119 (-54.0991, -24.4969) -> (-54.1926, -24.64) construction
  spline S72 degree 3 poles (-54.1926, -24.64) (-54.2057, -24.6092) (-54.2309, -24.5504) (-54.275, -24.4697) (-54.3239, -24.4012) (-54.3764, -24.3442) (-54.4323, -24.2991) (-54.4916, -24.2669) (-54.5538, -24.2465) (-54.5966, -24.2443) (-54.618, -24.2431) knots 0 0 0 0 0.162398 0.310626 0.445587 0.570114 0.685485 0.792558 0.896076 1 1 1 1 construction
  spline S73 degree 3 poles (-54.618, -24.2431) (-54.6299, -24.2434) (-54.6535, -24.244) (-54.6883, -24.2512) (-54.7226, -24.2616) (-54.7562, -24.2766) (-54.789, -24.2958) (-54.8214, -24.3189) (-54.8526, -24.3467) (-54.8941, -24.3896) (-54.9423, -24.4519) (-54.9923, -24.5379) (-55.0364, -24.6348) (-55.0724, -24.7428) (-55.1013, -24.8599) (-55.1221, -24.9846) (-55.1346, -25.1164) (-55.1362, -25.2067) (-55.137, -25.253) knots 0 0 0 0 0.028609 0.057304 0.085999 0.115554 0.146343 0.178161 0.21208 0.247572 0.322941 0.402722 0.48841 0.580947 0.678791 0.78097 0.887607 1 1 1 1 construction
  spline S74 degree 3 poles (-55.137, -25.253) (-55.1366, -25.2881) (-55.1358, -25.3569) (-55.1283, -25.4578) (-55.1172, -25.5542) (-55.1009, -25.6463) (-55.0801, -25.7339) (-55.0543, -25.8173) (-55.0238, -25.896) (-54.9894, -25.9697) (-54.951, -26.0365) (-54.9104, -26.0956) (-54.8666, -26.1453) (-54.8207, -26.1864) (-54.772, -26.2187) (-54.7204, -26.241) (-54.6666, -26.2559) (-54.6296, -26.2573) (-54.6109, -26.258) knots 0 0 0 0 0.085067 0.166468 0.244748 0.319783 0.392586 0.462695 0.530799 0.59673 0.659305 0.71706 0.76995 0.819293 0.865722 0.910695 0.954843 1 1 1 1 construction
  spline S75 degree 3 poles (-54.6109, -26.258) (-54.5904, -26.2569) (-54.5493, -26.2545) (-54.4895, -26.2346) (-54.4324, -26.2031) (-54.3786, -26.1585) (-54.3275, -26.1019) (-54.2789, -26.0331) (-54.2331, -25.9519) (-54.2065, -25.8924) (-54.1926, -25.8612) knots 0 0 0 0 0.100477 0.201249 0.306459 0.419158 0.54298 0.680156 0.831946 1 1 1 1 construction
  line L120 (-54.1926, -25.8612) -> (-54.0991, -26.0028) construction
  spline S76 degree 3 poles (-54.0991, -26.0028) (-54.1065, -26.0221) (-54.1212, -26.0601) (-54.1456, -26.1146) (-54.1706, -26.1662) (-54.1982, -26.2137) (-54.2259, -26.2588) (-54.2562, -26.2997) (-54.2872, -26.3377) (-54.3195, -26.3721) (-54.3533, -26.4025) (-54.3879, -26.4292) (-54.4237, -26.4514) (-54.4602, -26.4705) (-54.498, -26.4848) (-54.5369, -26.4947) (-54.5766, -26.5013) (-54.6036, -26.5019) (-54.6171, -26.5023) knots 0 0 0 0 0.081013 0.159304 0.233617 0.305251 0.37432 0.440667 0.504335 0.565969 0.625458 0.681844 0.736928 0.79009 0.842681 0.894758 0.947042 1 1 1 1 construction
  spline S77 degree 3 poles (-54.6171, -26.5023) (-54.6425, -26.501) (-54.6927, -26.4985) (-54.7656, -26.4779) (-54.8342, -26.4451) (-54.8985, -26.3988) (-54.9578, -26.339) (-55.0132, -26.2668) (-55.0645, -26.1816) (-55.0933, -26.1187) (-55.1084, -26.0858) knots 0 0 0 0 0.111248 0.21963 0.329364 0.443281 0.565014 0.697175 0.84133 1 1 1 1 construction
  spline S78 degree 3 poles (-55.1084, -26.0858) (-55.1206, -26.0559) (-55.1453, -25.9952) (-55.1752, -25.9) (-55.2019, -25.8007) (-55.2223, -25.6965) (-55.2395, -25.5881) (-55.2503, -25.4749) (-55.2579, -25.3574) (-55.2587, -25.2775) (-55.2592, -25.2367) knots 0 0 0 0 0.111525 0.226384 0.344601 0.4668 0.593002 0.723891 0.85931 1 1 1 1 construction
  spline S79 degree 3 poles (-55.2592, -25.2367) (-55.2586, -25.194) (-55.2576, -25.11) (-55.2488, -24.9868) (-55.2347, -24.8688) (-55.2148, -24.756) (-55.1888, -24.6484) (-55.1583, -24.5457) (-55.1207, -24.4485) (-55.0783, -24.3572) (-55.0319, -24.2738) (-54.9819, -24.2007) (-54.9286, -24.1389) (-54.8728, -24.0877) (-54.8136, -24.0477) (-54.7511, -24.0198) (-54.6858, -24.0022) (-54.6411, -24) (-54.6185, -23.9989) knots 0 0 0 0 0.08443 0.165585 0.24366 0.318878 0.391485 0.461966 0.530205 0.597027 0.660392 0.718361 0.771525 0.821065 0.867452 0.911834 0.955596 1 1 1 1 construction
  spline S80 degree 3 poles (-51.887, -26.5023) (-51.8961, -26.5019) (-51.9141, -26.5012) (-51.9406, -26.495) (-51.9668, -26.4863) (-51.9916, -26.4722) (-52.0166, -26.4558) (-52.0405, -26.4348) (-52.0639, -26.4105) (-52.0864, -26.3819) (-52.1086, -26.3492) (-52.1298, -26.3114) (-52.1507, -26.2687) (-52.1718, -26.2212) (-52.1916, -26.1683) (-52.2118, -26.1109) (-52.2306, -26.048) (-52.2427, -26.0044) (-52.249, -25.9818) knots 0 0 0 0 0.040342 0.080086 0.120502 0.162199 0.206453 0.253013 0.302946 0.356202 0.414164 0.478354 0.548449 0.625582 0.708712 0.79914 0.895844 1 1 1 1 construction